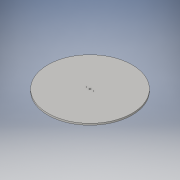
# Autodesk Inventor part: Zoetrope_Top
Saved by Autodesk Inventor 2016 (Build 200138000, 138)
## iProperties
Created: 2019-02-14
Part Number: Zoetrope_Top
Material: Generic
Document SubType Name: Modeling
Designer: student
Density: 1 g/cm^3
Appearance: Default
Author: student
Autodesk Inventor part; units mm, degrees
ref_plane "YZ Plane" through (0, 0, 0) normal (1, 0, 0) x (0, 1, 0)
ref_plane "XZ Plane" through (0, 0, 0) normal (0, 1, 0) x (-1, 0, 0)
ref_plane "XY Plane" through (0, 0, 0) normal (0, 0, 1) x (1, 0, 0)
sketch "Sketch1" plane through (0, 0, 0) normal (0, 1, 0) x (-1, 0, 0)
  circle A0 centre (0, 0) radius 114.3
  line L0 (0, 0) -> (80.8223, -80.8223)
  line L1 (0, 0) -> (114.3, 0)
  line L2 (0, 0) -> (80.8223, 80.8223)
  line L3 (0, 0) -> (114.3, 0) construction
  line L4 (0, 0) -> (-80.8223, -80.8223)
  line L5 (0, 0) -> (114.3, 0) construction
  line L6 (0, 0) -> (-80.8223, 80.8223)
  line L7 (0, 0) -> (114.3, 0) construction
  line L8 (0, 0) -> (105.5994, -43.7407) construction
  line L9 (0, 0) -> (114.3, 0) construction
  line L10 (0, 0) -> (43.7407, -105.5994) construction
  line L11 (0, 0) -> (114.3, 0) construction
  line L12 (0, 0) -> (105.5994, 43.7407) construction
  line L13 (0, 0) -> (43.7407, 105.5994) construction
  line L14 (0, 0) -> (-105.5994, 43.7407) construction
  line L15 (0, 0) -> (114.3, 0) construction
  line L16 (0, 0) -> (-43.7407, 105.5994) construction
  line L17 (0, 0) -> (-105.5994, -43.7407) construction
  line L18 (0, 0) -> (-43.7407, -105.5994) construction
  line L19 (0, 114.3) -> (0, 0)
  line L20 (0, 0) -> (-114.3, 0)
  line L21 (0, 0) -> (0, -114.3)
  line L22 (0, 0) -> (114.3, 0) construction
  circle A1 centre (0, 0) radius 2.2225
  line L23 (0, 0) -> (-9.525, 0)
  circle A2 centre (-9.525, 0) radius 0.9525
  line L24 (0, 0) -> (9.525, 0)
  circle A3 centre (9.525, 0) radius 0.9525
  line L25 (80.8223, -80.8223) -> (53.8815, -53.8815)
  line L26 (0, -114.3) -> (0, -76.2)
  dimension "d0" = 228.6
  dimension "d1" = 45
  dimension "d2" = 45
  dimension "d3" = 135
  dimension "d4" = 135
  dimension "d5" = 22.5
  dimension "d6" = 67.5
  dimension "d7" = 157.5
  dimension "d8" = 22.5
  dimension "d9" = 45
  dimension "d10" = 22.5
  dimension "d11" = 22.5
  dimension "d12" = 4.445
  dimension "d13" = 9.525
  dimension "d14" = 1.905
  dimension "d15" = 9.525
  dimension "d16" = 1.905
  constraints: 54 end point, 7 equal length, 7 horizontal, 5 point on line, 4 coincident, 3 centre point, 2 perpendicular, 1 collinear, 1 vertical, 17 other
  measures "d1" angle of L0 L1
  measures "d2" angle of L3 L2
  measures "d3" angle of L4 L5
  measures "d4" angle of L7 L6
  measures "d5" angle of L8 L9
  measures "d6" angle of L10 L11
  measures "d7" angle of L15 L14
  measures "d8" angle of L1 L12
  measures "d9" angle of L16 L13
  measures "d10" angle of L6 L16
  measures "d11" angle of L4 L18
  measures "d12" diameter of A1
  measures "d13" distance of L23.start L23.end
  measures "d14" diameter of A2
  measures "d15" distance of L23.start L24.end
  measures "d16" diameter of A3
extrude "Extrusion1" add sketch "Sketch1" along normal blind 4.572 contours L1 A3 A1 L2 A0 | A0 L0 A1 L1 A3 | L2 A1 L19 A0 | A0 L21 A1 L0 | L19 A1 L6 A0 | A0 L4 A1 L21 | L6 A1 L20 A2 A0 | A0 L20 A2 A1 L4
body "Solid1"
